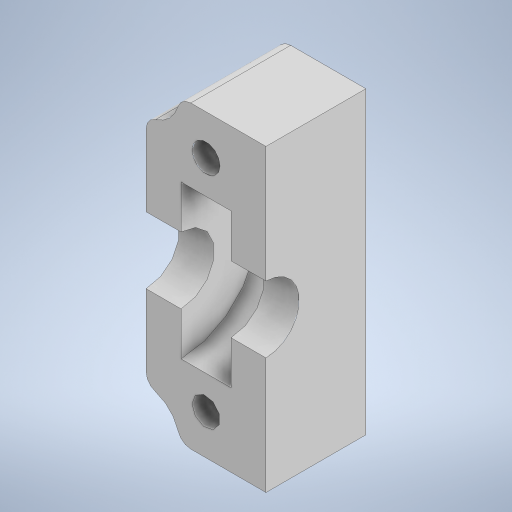
# Autodesk Inventor part: Bearing_holder_test_bottom
Saved by Autodesk Inventor 2024 (Build 280153000, 153)
## iProperties
Created: 2023-09-04
Part Number: Bearing_holder_test_bottom
Material: Generic
Document SubType Name: Modeling
Designer: Pintu
Density: 1 g/cm^3
Appearance: Default
Author: Pintu
Autodesk Inventor part; units mm, degrees
sketch "Sketch1" plane through (0, 0, 0) normal (0, 0, 1) x (1, 0, 0)
  line L0 (-55, 135) -> (55, 135)
  line L1 (55, 135) -> (55, -135)
  line L2 (55, -135) -> (-55, -135)
  line L3 (-55, -135) -> (-55, 135)
  line L4 (-55, 135) -> (55, -135) construction
  line L5 (55, 135) -> (-55, -135) construction
  line L6 (-45, -125) -> (-45, 132)
  line L7 (-45, 132) -> (45, 132)
  line L8 (45, 132) -> (45, -125)
  line L9 (45, -125) -> (-45, -125)
  line L10 (-55, 135) -> (-40, 135)
  line L11 (-40, 135) -> (-40, 120)
  line L12 (-40, 120) -> (-55, 120)
  line L13 (-55, 120) -> (-55, 135)
  line L14 (-55, -135) -> (-40, -135)
  line L15 (-40, -135) -> (-40, -120)
  line L16 (-40, -120) -> (-55, -120)
  line L17 (-55, -120) -> (-55, -135)
  line L18 (55, -135) -> (40, -135)
  line L19 (40, -135) -> (40, -120)
  line L20 (40, -120) -> (55, -120)
  line L21 (55, -120) -> (55, -135)
  line L22 (55, 135) -> (40, 135)
  line L23 (40, 135) -> (40, 120)
  line L24 (40, 120) -> (55, 120)
  line L25 (55, 120) -> (55, 135)
  point P0 (0, 0)
  point P1 (-40, -125)
  point P2 (-45, -120)
  point P3 (-45, 120)
  point P4 (-40, 132)
  point P5 (40, 132)
  point P6 (45, 120)
  point P7 (45, -120)
  point P8 (40, -125)
  dimension "d0" = 110
  dimension "d1" = 270
  dimension "d2" = 10
  dimension "d3" = 10
  dimension "d4" = 10
  dimension "d5" = 3
  dimension "shaft" = 15
  dimension "d7" = 15
  dimension "d8" = 15
  dimension "d9" = 15
  dimension "d10" = 15
  dimension "d11" = 15
  dimension "d12" = 15
  dimension "d13" = 15
  constraints: 52 end point, 12 parallel, 6 perpendicular, 5 horizontal, 2 midpoint, 1 vertical
  measures "d0" distance of L1.end L2.end
  measures "d1" distance of L0.end L1.end
  measures "d2" distance between parallel lines of L1 L8
  measures "d3" distance between parallel lines of L3 L6
  measures "d4" distance between parallel lines of L2 L9
  measures "d5" distance between parallel lines of L0 L7
  measures "shaft" distance of L11.end L12.end
  measures "d7" distance of L10.end L11.end
  measures "d8" distance of L16.end L15.end
  measures "d9" distance of L15.end L14.end
  measures "d10" distance of L19.end L20.end
  measures "d11" distance of L18.end L19.end
  measures "d12" distance of L24.end L23.end
  measures "d13" distance of L23.end L22.end
extrude "Extrusion1" add sketch "Sketch1" along normal blind 30 contours L0 L11 L7 L6 L12 L3 | L0 L23 L7 L11 | L12 L6 L16 L3 | L0 L1 L24 L8 L7 L23 | L11 L12 L6 L7 | L16 L6 L9 L15 L2 L3 | L7 L8 L24 L23 | L16 L15 L9 L6 | L1 L20 L8 L24 | L15 L9 L19 L2 | L1 L2 L19 L9 L8 L20 | L8 L9 L19 L20
sketch "Sketch2" plane through (0, 0, 30) normal (0, 0, 1) x (1, 0, 0)
  line L0 (-55, 135) -> (-55, -135) projected
  line L1 (-55, -70) -> (-37, -70)
  line L2 (-37, -70) -> (-37, -115)
  line L3 (-37, -115) -> (-55, -115)
  line L4 (-55, -115) -> (-55, -70)
  line L5 (-55, -135) -> (55, -135) projected
  line L6 (55, -135) -> (55, 135) projected
  line L7 (55, -115) -> (37, -115)
  line L8 (37, -115) -> (37, -70)
  line L9 (37, -70) -> (55, -70)
  line L10 (55, -70) -> (55, -115)
  point P0 (0, 0)
  dimension "wheelHolderBreath" = 18
  dimension "wheelHolderlength" = 45
  dimension "DistanceWH" = 20
  dimension "d19" = 18
  dimension "d20" = 45
  dimension "d21" = 20
  constraints: 16 end point, 4 parallel, 2 horizontal, 2 perpendicular, 2 point on line
  measures "wheelHolderBreath" distance of L2.end L3.end
  measures "wheelHolderlength" distance of L1.end L2.end
  measures "DistanceWH" distance between parallel lines of L5 L3
  measures "d19" distance of L8.end L9.end
  measures "d20" distance of L7.end L8.end
  measures "d21" distance between parallel lines of L5 L7
extrude "Extrusion2" add sketch "Sketch2" against normal blind 30
fillet "Fillet1" radius 5 4 edges at (-37, -70, 15) (-37, -115, 15) (37, -70, 15) (37, -115, 15) inverted yes
fillet "Fillet2" radius 2 8 edges at (-42, -70, 15) (-42, -115, 15) (42, -115, 15) (42, -70, 15) (-37, -75, 15) (-37, -110, 15) (37, -110, 15) (37, -75, 15)
extrude "Extrusion3" cut sketch "Sketch2" against normal blind 15
ref_plane "Work Plane1" through (-46, -108.2918, 0) normal (1, 0, 0) x (0, 0, -1)
sketch "Sketch3" plane through (-46, -108.2918, 0) normal (1, 0, 0) x (0, 0, -1)
  line L0 (-30, -6.7082) -> (-15, -6.7082) projected
  line L1 (-15, -6.7082) -> (-15, 38.2918) projected
  line L2 (-15, 38.2918) -> (-30, 38.2918) projected
  line L3 (-30, 243.2918) -> (-30, 38.2918) projected
  line L4 (0, 243.2918) -> (-30, 243.2918) projected
  line L5 (0, 243.2918) -> (0, -26.7082) projected
  line L6 (0, -26.7082) -> (-30, -26.7082) projected
  line L7 (-30, -6.7082) -> (-30, -26.7082) projected
  line L8 (-15, 38.2918) -> (-30, 38.2918) projected
  line L9 (-30, -6.7082) -> (-15, -6.7082) projected
  line L10 (-15, -6.7082) -> (-15, 38.2918) projected
  circle A0 centre (-15, 15.7918) radius 11.5
  point P0 (0, 108.2918)
  dimension "d28" = 23
  constraints: 1 centre point, 1 midpoint
  measures "d28" diameter of A0
extrude "Extrusion4" cut sketch "Sketch3" along normal mid plane 7.5 contours A0 L1 | L1 A0
ref_plane "Work Plane2" through (-39.625, -108.2918, 0) normal (1, 0, 0) x (0, 0, -1)
sketch "Sketch4" plane through (-39.625, -108.2918, 0) normal (1, 0, 0) x (0, 0, -1)
  line L0 (-15, 27.2918) -> (-15, 4.2918) projected
  line L1 (-15, 27.2918) -> (-15, 4.2918) projected
  arc A0 (-15, 4.2918) -> (-15, 27.2918) centre (-15, 15.7918) ccw projected
  circle A1 centre (-15, 15.7918) radius 5
  point P0 (0, 108.2918)
  dimension "d31" = 10
  constraints: 1 centre point, 1 coincident
  measures "d31" diameter of A1
extrude "Extrusion5" cut sketch "Sketch4" along normal mid plane 50 contours A1 L0 | L0 A1
sketch "Sketch5" plane through (0, 0, 0) normal (0, 0, -1) x (-1, 0, 0)
  line L0 (55, 135) -> (55, -135) projected
  line L1 (45, -70) -> (43.7082, -70) projected
  point P0 (0, 0)
  point P1 (46, -76)
  dimension "d36" = 9
  dimension "d37" = 6
  measures "d36" distance from line of L0 point (46, -76)
  measures "d37" distance from line of L1 point (46, -76)
hole "Hole1" at (-46, -76, 0) direction (0, 0, 1) diameter 4.2 end through all counterbore diameter 7.5 counterbore depth 4.6 clearance for "Socket Head Cap Screw ISO 4762" size "M4" standard "ISO"
sketch "Sketch6" plane through (0, 0, 0) normal (0, 0, -1) x (-1, 0, 0)
  line L0 (37, -76.7082) -> (37, -108.2918) projected
  line L1 (43.7082, -115) -> (45, -115) projected
  point P0 (0, 0)
  point P1 (46, -109)
  dimension "d45" = 9
  dimension "d46" = 6
  measures "d45" distance from line of L0 point (46, -109)
  measures "d46" distance from line of L1 point (46, -109)
hole "Hole2" at (-46, -109, 0) direction (0, 0, 1) diameter 4.2 end through all counterbore diameter 7.5 counterbore depth 4.6 clearance for "Socket Head Cap Screw ISO 4762" size "M4" standard "ISO"
ref_plane "Work Plane3" through (0, -135, 0) normal (1, 0, 0) x (0, 0, -1)
mirror "Mirror1" about plane through (0, -135, 0) normal (1, 0, 0) of "Extrusion3", "Hole1", "Hole2", "Extrusion5", "Extrusion4"
sketch "Sketch7" plane through (0, 0, 0) normal (0, 0, -1) x (-1, 0, 0)
  circle A0 centre (-46, -109) radius 3.75 projected
  circle A1 centre (-46, -76) radius 3.75 projected
  circle A2 centre (46, -109) radius 3.75 projected
  circle A3 centre (46, -76) radius 3.75 projected
  arc A4 (-37, -76.7082) -> (-38.4286, -74.7916) centre (-39, -76.7082) ccw projected
  arc A5 (-41.7916, -71.4286) -> (-38.4286, -74.7916) centre (-37, -70) ccw projected
  arc A6 (-41.7916, -71.4286) -> (-43.7082, -70) centre (-43.7082, -72) ccw projected
  line L0 (-43.7082, -70) -> (-45, -70) projected
  line L1 (-45, 120) -> (-45, -70) projected
  line L2 (-40, 120) -> (-45, 120) projected
  line L3 (-40, 132) -> (-40, 120) projected
  line L4 (40, 132) -> (-40, 132) projected
  line L5 (40, 120) -> (40, 132) projected
  line L6 (45, 120) -> (40, 120) projected
  line L7 (45, -70) -> (45, 120) projected
  line L8 (45, -70) -> (43.7082, -70) projected
  arc A7 (43.7082, -70) -> (41.7916, -71.4286) centre (43.7082, -72) ccw projected
  arc A8 (38.4286, -74.7916) -> (41.7916, -71.4286) centre (37, -70) ccw projected
  arc A9 (38.4286, -74.7916) -> (37, -76.7082) centre (39, -76.7082) ccw projected
  line L9 (37, -76.7082) -> (37, -108.2918) projected
  arc A10 (37, -108.2918) -> (38.4286, -110.2084) centre (39, -108.2918) ccw projected
  arc A11 (41.7916, -113.5714) -> (38.4286, -110.2084) centre (37, -115) ccw projected
  arc A12 (41.7916, -113.5714) -> (43.7082, -115) centre (43.7082, -113) ccw projected
  line L10 (43.7082, -115) -> (45, -115) projected
  line L11 (45, -120) -> (45, -115) projected
  line L12 (40, -120) -> (45, -120) projected
  line L13 (40, -125) -> (40, -120) projected
  line L14 (-40, -125) -> (40, -125) projected
  line L15 (-40, -120) -> (-40, -125) projected
  line L16 (-45, -120) -> (-40, -120) projected
  line L17 (-45, -115) -> (-45, -120) projected
  line L18 (-45, -115) -> (-43.7082, -115) projected
  arc A13 (-43.7082, -115) -> (-41.7916, -113.5714) centre (-43.7082, -113) ccw projected
  arc A14 (-38.4286, -110.2084) -> (-41.7916, -113.5714) centre (-37, -115) ccw projected
  arc A15 (-38.4286, -110.2084) -> (-37, -108.2918) centre (-39, -108.2918) ccw projected
  line L19 (-37, -108.2918) -> (-37, -76.7082) projected
  line L20 (-55, -135) -> (-55, 135) projected
  line L21 (55, -135) -> (-55, -135) projected
  line L22 (55, 135) -> (55, -135) projected
  line L23 (-55, 135) -> (55, 135) projected
  line L24 (-55, 85) -> (55, 85)
  line L25 (55, 85) -> (55, 75)
  line L26 (55, 75) -> (-55, 75)
  line L27 (-55, 75) -> (-55, 85)
  point P0 (0, 0)
  point P1 (-55, 75)
  dimension "d54" = 10
  dimension "d55" = 220
  constraints: 8 end point, 2 parallel, 2 perpendicular, 2 point on line
  measures "d54" distance of L24.end L25.end
  measures "d55" distance between parallel lines of L21 L24
extrude "Extrusion7" add sketch "Sketch7" against normal blind 30 contours L26 L20 L24 L1 | L1 L24 L7 L26 | L7 L24 L22 L26
sketch "Sketch12" plane through (0, 0, 30) normal (0, 0, 1) x (1, 0, 0)
  line L0 (55, -115) -> (45, -115) projected
  line L1 (45, -115) -> (45, -120) projected
  line L2 (45, -120) -> (40, -120) projected
  line L3 (40, -120) -> (40, -125) projected
  line L4 (40, -125) -> (-40, -125) projected
  line L5 (-40, -125) -> (-40, -120) projected
  line L6 (-40, -120) -> (-45, -120) projected
  line L7 (-45, -120) -> (-45, -115) projected
  line L8 (-45, -115) -> (-55, -115) projected
  line L9 (-55, -115) -> (-55, -135) projected
  line L10 (-55, -135) -> (55, -135) projected
  line L11 (55, -135) -> (55, -115) projected
  point P0 (0, 0)
extrude "Extrusion11" cut sketch "Sketch12" against normal blind 30
sketch "Sketch13" plane through (0, 0, 30) normal (0, 0, 1) x (1, 0, 0)
  line L0 (45, 75) -> (45, -70) projected
  line L1 (45, 75) -> (45, -70) projected
  line L2 (45, -70) -> (55, -70) projected
  line L3 (55, -70) -> (55, 135) projected
  line L4 (55, 135) -> (-55, 135) projected
  line L5 (-55, 135) -> (-55, -70) projected
  line L6 (-55, -70) -> (-45, -70) projected
  line L7 (-45, -70) -> (-45, 75) projected
  line L8 (-45, 75) -> (45, 75) projected
  line L9 (45, 85) -> (-45, 85) projected
  line L10 (-45, 85) -> (-45, 120) projected
  line L11 (-45, 120) -> (-40, 120) projected
  line L12 (-40, 120) -> (-40, 132) projected
  line L13 (-40, 132) -> (40, 132) projected
  line L14 (40, 132) -> (40, 120) projected
  line L15 (40, 120) -> (45, 120) projected
  line L16 (45, 120) -> (45, 85) projected
  point P0 (0, 0)
  point P1 (45, -70)
extrude "Extrusion12" cut sketch "Sketch13" against normal blind 30
sketch "Sketch14" plane through (0, 0, 0) normal (0, 0, -1) x (-1, 0, 0)
  circle A0 centre (46, -76) radius 3.75 projected
  circle A1 centre (46, -109) radius 3.75 projected
  line L0 (55, -70) -> (43.7082, -70) projected
  arc A2 (43.7082, -70) -> (41.7916, -71.4286) centre (43.7082, -72) ccw projected
  arc A3 (38.4286, -74.7916) -> (41.7916, -71.4286) centre (37, -70) ccw projected
  arc A4 (38.4286, -74.7916) -> (37, -76.7082) centre (39, -76.7082) ccw projected
  line L1 (37, -76.7082) -> (37, -108.2918) projected
  arc A5 (37, -108.2918) -> (38.4286, -110.2084) centre (39, -108.2918) ccw projected
  arc A6 (41.7916, -113.5714) -> (38.4286, -110.2084) centre (37, -115) ccw projected
  arc A7 (41.7916, -113.5714) -> (43.7082, -115) centre (43.7082, -113) ccw projected
  line L2 (43.7082, -115) -> (55, -115) projected
  line L3 (55, -70) -> (55, -115) projected
  circle A8 centre (46, -109) radius 3.75 projected
  circle A9 centre (46, -109) radius 2.1 projected
  circle A10 centre (46, -76) radius 3.75 projected
  circle A11 centre (46, -76) radius 2.1 projected
  point P0 (0, 0)
extrude "Extrusion13" cut sketch "Sketch14" against normal blind 30 contours A0 | A1 | L3 L2 A7 A6 A5 L1 A4 A3 A2 L0 | A9
equation "\"d7\" = shaft"
equation "\"d8\" = shaft"
equation "\"d9\" = shaft"
equation "\"d10\" = shaft"
equation "\"d11\" = shaft"
equation "\"d12\" = shaft"
equation "\"d13\" = shaft"
equation "\"d19\" = wheelHolderBreath"
equation "\"d20\" = wheelHolderlength"
equation "\"d21\" = DistanceWH"
body "Solid1"
